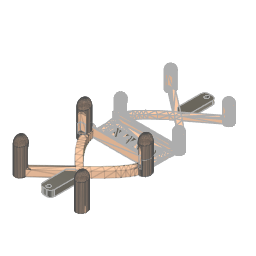
nano_breadboard_heart rate_holder (Autodesk Fusion 360 design; units mm, degrees)
Autodesk Fusion 360 part; units mm, degrees
other "Base Mesh Feature1"
other "Body->Comp1"
sketch "Sketch1" plane through (0, 0, 0) normal (0, 0, 1) x (1, 0, 0)
  circle A0 centre (-16.8045, -1.788) radius 1 construction
  line L0 (-12.3045, -1.288) -> (-21.3045, -1.288) construction
  line L1 (-21.3045, -1.288) -> (-21.3045, -2.288) construction
  line L2 (-21.3045, -2.288) -> (-12.3045, -2.288) construction
  line L3 (-12.3045, -2.288) -> (-12.3045, -1.288) construction
  line L4 (-12.3045, -1.288) -> (-21.3045, -2.288) construction
  line L5 (-21.3045, -1.288) -> (-12.3045, -2.288) construction
  line L6 (-16.8045, -1.788) -> (-21.3045, -1.788) construction
  line L7 (-16.8045, -1.788) -> (-12.3045, -1.788) construction
  line L8 (-21.3045, -1.788) -> (-12.3045, -1.788)
  line L9 (-12.3045, -1.788) -> (-12.3045, 22.212)
  line L10 (-12.3045, 22.212) -> (-21.3045, 22.212)
  line L11 (-21.3045, 22.212) -> (-21.3045, -1.788)
  point P0 (-16.8045, -1.788)
  dimension "d1" = 2
  dimension "d2" = 9
  dimension "d3" = 1
  dimension "d4" = 9
  dimension "d5" = 24
  constraint horizontal L0
  constraint perpendicular L0 L1
  constraint parallel L0 L2
  constraint parallel L1 L3
  constraint coincident L4 P0
  constraint coincident L5 P0
  constraint coincident P0 A0.centre
  constraint midpoint L1 L6.end
  constraint midpoint L3 L7.end
  constraint horizontal L8
  constraint vertical L9
  constraint horizontal L10
  constraint vertical L11
  measures "d1" diameter of A0
  measures "d2" distance of L1.end L2.end
  measures "d3" distance of L0.end L1.end
  measures "d4" distance of L6.end L7.end
  measures "d5" distance of L6.end L10.end
extrude "Extrude1" add sketch "Sketch1" along normal blind 3 makes body 1
fillet "Fillet1" radius 3 2 edges at (-21.3045, 22.212, 1.5) (-12.3045, 22.212, 1.5) on bodies 1
chamfer "Chamfer1" distance 3.4 angle 45 2 edges at (-21.3045, -1.788, 1.5) (-12.3045, -1.788, 1.5) on bodies 1
sketch "Sketch2" plane through (0, 0, 3) normal (0, 0, 1) x (-1, 0, 0)
  line L0 (15.7045, 1.788) -> (12.3045, -1.612)
  line L1 (12.3045, -1.612) -> (12.3045, -19.212)
  arc A0 (12.3045, -19.212) -> (15.3045, -22.212) centre (15.3045, -19.212) ccw
  line L2 (15.3045, -22.212) -> (18.3045, -22.212)
  arc A1 (18.3045, -22.212) -> (21.3045, -19.212) centre (18.3045, -19.212) ccw
  line L3 (21.3045, -19.212) -> (21.3045, -1.612)
  line L4 (21.3045, -1.612) -> (17.9045, 1.788)
  line L5 (17.9045, 1.788) -> (15.7045, 1.788)
  circle A2 centre (16.8045, -19.27) radius 1.5
  dimension "d11" = 3
  measures "d11" diameter of A2
extrude "Extrude2" cut sketch "Sketch2" against normal up to surface (3 mm away) contours A2 bodies 1
sketch "Sketch3" plane through (0, 0, 0) normal (0, 0, 1) x (1, 0, 0)
  line L0 (-33.5, -33.5) -> (0, -33.5)
  line L1 (0, -33.5) -> (0, -42.5)
  line L2 (0, -42.5) -> (-33.5, -42.5)
  line L3 (-33.5, -42.5) -> (-33.5, -33.5)
  constraint horizontal L0
  constraint vertical L1
  constraint horizontal L2
  constraint vertical L3
extrude "Extrude3" add sketch "Sketch3" along normal blind 1.5 separate body makes body 2
sketch "Sketch4" plane through (0, 0, 0) normal (0, 0, 1) x (1, 0, 0)
copy_body "CutPasteBodies1" bodies 1 2 removing the originals makes body 3 makes body 4 in component "Support_Nano__mini_bread_board"
sketch "Sketch1 (2)" plane through (0, 0, 0) normal (0, 1, 0) x (1, 0, 0) in component "Support_Nano__mini_bread_board"
sketch "Sketch2 (2)" plane through (0, 0, 0) normal (0, 0, 1) x (1, 0, 0) in component "Support_Nano__mini_bread_board"
  line L0 (-39.316, -48.7899) -> (5.684, -48.7899)
  line L1 (-12.316, -48.2899) -> (-21.316, -48.2899) construction
  line L2 (-21.316, -48.2899) -> (-21.316, -49.2899) construction
  line L3 (-21.316, -49.2899) -> (-12.316, -49.2899) construction
  line L4 (-12.316, -49.2899) -> (-12.316, -48.2899) construction
  line L5 (-12.316, -48.2899) -> (-21.316, -49.2899) construction
  line L6 (-21.316, -48.2899) -> (-12.316, -49.2899) construction
  line L7 (-16.816, -48.7899) -> (-21.316, -48.7899) construction
  line L8 (-16.816, -48.7899) -> (-12.316, -48.7899) construction
  line L9 (-21.316, -48.7899) -> (-12.316, -48.7899)
  line L10 (-12.316, -48.7899) -> (-12.316, -56.7899)
  line L11 (-12.316, -56.7899) -> (-21.316, -56.7899)
  line L12 (-21.316, -56.7899) -> (-21.316, -48.7899)
  point P0 (-16.816, -48.7899)
  dimension "d16" = 9
  dimension "d17" = 1
  dimension "d18" = 9
  dimension "d19" = 8
  constraint horizontal L0
  constraint horizontal L1
  constraint perpendicular L1 L2
  constraint parallel L1 L3
  constraint parallel L2 L4
  constraint coincident L5 P0
  constraint coincident L6 P0
  constraint midpoint L0 P0
  constraint coincident P0 L7.start
  constraint midpoint L2 L7.end
  constraint midpoint L4 L8.end
  constraint horizontal L9
  constraint vertical L10
  constraint horizontal L11
  constraint vertical L12
  measures "d16" distance of L2.end L3.end
  measures "d17" distance of L1.end L2.end
  measures "d18" distance of L7.end L8.end
  measures "d19" distance of L7.end L11.end
sketch "Sketch3 (2)" plane through (0, 0, 3) normal (0, 0, 1) x (-1, 0, 0) in component "Support_Nano__mini_bread_board"
  line L0 (21.316, 48.7899) -> (21.316, 56.7899)
  line L1 (21.316, 56.7899) -> (12.316, 56.7899)
  line L2 (12.316, 56.7899) -> (12.316, 48.7899)
  line L3 (12.316, 48.7899) -> (21.316, 48.7899)
  circle A0 centre (16.816, 52.7899) radius 1.5
  dimension "d23" = 3
  measures "d23" diameter of A0
sketch "Sketch4 (2)" plane through (0, 0, 0) normal (0, 0, 1) x (1, 0, 0) in component "Support_Nano__mini_bread_board"
  circle A0 centre (5.1944, -51.2544) radius 3.3823
sketch "Sketch5" plane through (0, 0, 7) normal (0, 0, 1) x (-1, 0, 0) in component "Support_Nano__mini_bread_board"
  circle A0 centre (-5.1762, 51.1414) radius 3.3823
  line L0 (-2.2251, 52.7939) -> (-6.0876, 52.7939)
  line L1 (-6.0876, 52.7939) -> (-6.0876, 54.4955)
  line L2 (-6.0876, 54.4955) -> (-2.9609, 54.6946)
  line L3 (-2.9609, 54.6946) -> (-2.2251, 52.7939)
  constraint coincident A0 L0.start
  constraint horizontal L0
  constraint perpendicular L0 L1
other "CopyPasteMeshes3" in component "Support_Nano__mini_bread_board"
other "Modify2" in component "Support_Nano__mini_bread_board"
other "Body->Comp2" in component "Support_Nano__mini_bread_board"
other "Base Mesh Feature1'" in component "Support_Nano__mini_bread_board (1)"
other "Scale1" in component "Support_Nano__mini_bread_board (1)"
other "Modify1" in component "Support_Nano__mini_bread_board (1)"
copy_body "CopyPasteBodies3" bodies 3 makes body 5 in component "Support_Nano__mini_bread_board"
move_body "Move2" bodies 5 to x (-1, 0, 0) y (0, -1, 0) z (0, 0, 1) at (-33.4671, -76.6961, 0) in component "Support_Nano__mini_bread_board"
move_face "OffsetFaces1" offset 1.65 1 faces at (-16.6999, -83.6955, 3) on bodies 5 in component "Support_Nano__mini_bread_board"
sketch "Sketch1 (3)" plane through (0, 0, 0) normal (0, 0, 1) x (1, 0, 0) in component "Support_Nano__mini_bread_board (1)"
  line L0 (6.6333, -40.669) -> (6.286, -49.5717)
  ellipse E0 centre (6.4597, -45.1203) end of major axis (6.286, -49.5717) minor radius 3.546
  line L1 (6.6333, -40.669) -> (6.286, -49.5717)
  line L2 (2.9163, -44.9821) -> (10.003, -45.2585)
  constraint midpoint L0 E0.centre
  constraint coincident L0.start E0
  constraint coincident E0 L2.start
  constraint coincident E0 L2.end
extrude "Extrude1'" add sketch "Sketch1 (3)" along normal blind 11 separate body makes body 6 in component "Support_Nano__mini_bread_board (1)"
sketch "Sketch2 (3)" plane through (0, 0, 0) normal (0, 0, 1) x (1, 0, 0) in component "Support_Nano__mini_bread_board (1)"
  line L0 (-40.4124, -40.6626) -> (-40.4124, -49.568)
  ellipse E0 centre (-40.4124, -45.1153) end of major axis (-40.4124, -49.568) minor radius 3.5014
  line L1 (-40.4124, -40.6626) -> (-40.4124, -49.568)
  line L2 (-43.9138, -45.1153) -> (-36.911, -45.1153)
  constraint vertical L0
  constraint midpoint L0 E0.centre
  constraint coincident L0.start E0
  constraint coincident E0 L2.start
  constraint coincident E0 L2.end
extrude "Extrude2'" add sketch "Sketch2 (3)" along normal blind 10.5 separate body makes body 7 in component "Support_Nano__mini_bread_board (1)"
sketch "Sketch3 (3)" plane through (0, 0, 11) normal (0, 0, 1) x (-1, 0, 0) in component "Support_Nano__mini_bread_board (1)"
  ellipse E0 centre (-6.4597, 45.1203) end of major axis (-6.286, 49.5717) minor radius 3.546
  line L0 (-3.1253, 46.9904) -> (-7.3402, 46.9904)
  line L1 (-7.3402, 46.9904) -> (-7.3402, 49.5254)
  line L2 (-7.3402, 49.5254) -> (-4.8438, 50.6121)
  line L3 (-4.8438, 50.6121) -> (-2.7959, 47.482)
  line L4 (-2.7959, 47.482) -> (-3.1253, 46.9904)
  constraint horizontal L0
  constraint perpendicular L0 L1
extrude "Extrude3'" cut sketch "Sketch3 (3)" against normal blind 6.4 contours E0 L0 L1 picked at (-4.6808, 47.2003) bodies 6 in component "Support_Nano__mini_bread_board (1)"
sketch "Sketch4 (3)" plane through (0, 0, 10.5) normal (0, 0, 1) x (-1, 0, 0) in component "Support_Nano__mini_bread_board (1)"
  ellipse E0 centre (40.4124, 45.1153) end of major axis (40.4124, 49.568) minor radius 3.5014
  line L0 (41.2268, 46.9535) -> (37.1082, 46.9535)
  line L1 (37.1082, 46.9535) -> (37.2281, 50.274)
  line L2 (37.2281, 50.274) -> (41.2526, 50.8471)
  line L3 (41.2526, 50.8471) -> (41.2268, 46.9535)
  constraint horizontal L0
extrude "Extrude4" cut sketch "Sketch4 (3)" against normal blind 6 contours E0 L0 L3 picked at (38.8444, 47.5487) bodies 7 in component "Support_Nano__mini_bread_board (1)"
other "Modify3" in component "Support_Nano__mini_bread_board"
move_body "Move3" bodies 5 to x (1, 0, 0) y (0, 1, 0) z (0, 0, 1) at (0, -6, 0) in component "Support_Nano__mini_bread_board"
move_body "Move4" bodies 5 to x (1, 0, 0) y (0, 1, 0) z (0, 0, 1) at (0, 1, 0) in component "Support_Nano__mini_bread_board"
move_body "Move5" bodies 4 to x (1, 0, 0) y (0, 1, 0) z (0, 0, 1) at (0, 1, 0) in component "Support_Nano__mini_bread_board"
component "Support_Nano__mini_bread_board" placed x (1, 0, 0) y (0, 1, 0) z (0, 0, 1) at (0, 0, 0)
component "Support_Nano__mini_bread_board (1)" placed x (1, 0, 0) y (0, 1, 0) z (0, 0, 1) at (0.2018, -5.3945, 0) in component "Support_Nano__mini_bread_board"
